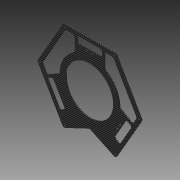
# Autodesk Inventor part: Bottom Plate
Saved by Autodesk Inventor 2015 (Build 190159000, 159)
## iProperties
Created: 2016-10-01
Part Number: Bottom Plate
Material: Generic
Document SubType Name: Modeling
Designer: James Yelland
Density: 1 g/cm^3
Appearance: Default
Author: James Yelland
Autodesk Inventor part; units mm, degrees
ref_plane "YZ Plane" through (0, 0, 0) normal (1, 0, 0) x (0, 1, 0)
ref_plane "XZ Plane" through (0, 0, 0) normal (0, 1, 0) x (-1, 0, 0)
ref_plane "XY Plane" through (0, 0, 0) normal (0, 0, 1) x (1, 0, 0)
sketch "Sketch1" plane through (0, 0, 0) normal (0, 1, 0) x (-1, 0, 0)
  line L0 (72.6878, -41.9663) -> (62.1878, -60.1529)
  line L1 (72.6878, -41.9663) -> (83.1878, -23.7798)
  line L2 (81.7237, -18.3157) -> (77.3936, -15.8157)
  line L3 (71.9295, -17.2797) -> (50.9295, -53.6529)
  line L4 (52.3936, -59.117) -> (56.7237, -61.617)
  arc A0 (56.7237, -61.617) -> (62.1878, -60.1529) centre (58.7237, -58.1529) ccw
  arc A1 (50.9295, -53.6529) -> (52.3936, -59.117) centre (54.3936, -55.6529) ccw
  arc A2 (77.3936, -15.8157) -> (71.9295, -17.2797) centre (75.3936, -19.2798) ccw
  arc A3 (83.1878, -23.7798) -> (81.7237, -18.3157) centre (79.7237, -21.7798) ccw
  line L5 (55.5994, -35.5644) -> (57.3314, -36.5644)
  line L6 (57.3314, -36.5644) -> (54.8314, -40.8945)
  line L7 (53.0994, -39.8945) -> (55.5994, -35.5644)
  line L8 (54.8314, -40.8945) -> (53.0994, -39.8945)
  line L9 (61.0994, -26.0381) -> (58.5994, -30.3683)
  line L10 (60.3314, -31.3683) -> (62.8314, -27.0381)
  line L11 (58.5994, -30.3683) -> (60.3314, -31.3683)
  line L12 (62.8314, -27.0381) -> (61.0994, -26.0381)
  line L13 (0, 83.9327) -> (21, 83.9327)
  line L14 (0, 83.9327) -> (-21, 83.9327)
  line L15 (-25, 79.9327) -> (-25, 74.9327)
  line L16 (-21, 70.9327) -> (20.9998, 70.9327)
  line L17 (25, 74.9327) -> (25, 79.9327)
  arc A4 (25, 79.9327) -> (21, 83.9327) centre (21, 79.9327) ccw
  arc A5 (20.9998, 70.9327) -> (25, 74.9327) centre (21, 74.9327) ccw
  arc A6 (-25, 74.9327) -> (-21, 70.9327) centre (-21, 74.9327) ccw
  arc A7 (-21, 83.9327) -> (-25, 79.9327) centre (-21, 79.9327) ccw
  line L18 (3, 65.9327) -> (3, 67.9327)
  line L19 (8, 65.9327) -> (3, 65.9327)
  line L20 (8, 67.9327) -> (8, 65.9327)
  line L21 (3, 67.9327) -> (8, 67.9327)
  line L22 (-8, 67.9327) -> (-8, 65.9327)
  line L23 (-8, 65.9327) -> (-3, 65.9327)
  line L24 (-3, 65.9327) -> (-3, 67.9327)
  line L25 (-3, 67.9327) -> (-8, 67.9327)
  line L26 (-72.6878, -41.9663) -> (-83.1878, -23.7798)
  line L27 (-72.6878, -41.9663) -> (-62.1878, -60.1529)
  line L28 (-56.7237, -61.617) -> (-52.3936, -59.117)
  line L29 (-50.9295, -53.6529) -> (-71.9294, -17.28)
  line L30 (-77.3936, -15.8157) -> (-81.7237, -18.3157)
  arc A8 (-81.7237, -18.3157) -> (-83.1878, -23.7798) centre (-79.7237, -21.7798) ccw
  arc A9 (-71.9294, -17.28) -> (-77.3936, -15.8157) centre (-75.3936, -19.2798) ccw
  arc A10 (-52.3936, -59.117) -> (-50.9295, -53.6529) centre (-54.3936, -55.6529) ccw
  arc A11 (-62.1878, -60.1529) -> (-56.7237, -61.617) centre (-58.7237, -58.1529) ccw
  line L31 (-58.5994, -30.3683) -> (-60.3314, -31.3683)
  line L32 (-61.0994, -26.0381) -> (-58.5994, -30.3683)
  line L33 (-62.8314, -27.0381) -> (-61.0994, -26.0381)
  line L34 (-60.3314, -31.3683) -> (-62.8314, -27.0381)
  line L35 (-54.8314, -40.8945) -> (-53.0994, -39.8945)
  line L36 (-53.0994, -39.8945) -> (-55.5994, -35.5644)
  line L37 (-55.5994, -35.5644) -> (-57.3314, -36.5644)
  line L38 (-57.3314, -36.5644) -> (-54.8314, -40.8945)
  line L39 (103.5566, -2.5) -> (54.8095, -86.9325)
  line L40 (-54.8095, -86.9325) -> (-103.5566, -2.5)
  line L41 (-103.5566, 2.5) -> (-53.9434, 88.4327)
  line L42 (-49.6132, 90.9327) -> (49.6132, 90.9327)
  line L43 (53.9434, 88.4327) -> (103.5566, 2.5)
  line L44 (2.1497, -66.9563) -> (48.3297, -88.9468)
  line L45 (-2.1497, -66.9563) -> (-48.3297, -88.9468)
  arc A12 (48.3297, -88.9468) -> (54.8095, -86.9325) centre (50.4794, -84.4325) ccw
  arc A13 (2.1497, -66.9563) -> (-2.1497, -66.9563) centre (0, -71.4706) ccw
  arc A14 (-54.8095, -86.9325) -> (-48.3297, -88.9468) centre (-50.4794, -84.4325) ccw
  arc A15 (-103.5566, 2.5) -> (-103.5566, -2.5) centre (-99.2265, 0) ccw
  arc A16 (-49.6132, 90.9327) -> (-53.9434, 88.4327) centre (-49.6132, 85.9327) ccw
  arc A17 (53.9434, 88.4327) -> (49.6132, 90.9327) centre (49.6132, 85.9327) ccw
  arc A18 (103.5566, -2.5) -> (103.5566, 2.5) centre (99.2265, 0) ccw
  circle A19 centre (49.6132, 85.9327) radius 1.6
  circle A20 centre (-49.6132, 85.9327) radius 1.6
  circle A21 centre (-99.2265, 0) radius 1.6
  circle A22 centre (99.2265, 0) radius 1.6
  line L46 (48.9434, 79.7724) -> (93.5566, 2.5)
  line L47 (-35, 82.2724) -> (-44.6132, 82.2724)
  line L48 (35, 82.2724) -> (44.6132, 82.2724)
  arc A23 (35, 82.2724) -> (30, 77.2724) centre (35, 77.2724) ccw
  arc A24 (-30, 77.2724) -> (-35, 82.2724) centre (-35, 77.2724) ccw
  arc A25 (48.9434, 79.7724) -> (44.6132, 82.2724) centre (44.6132, 77.2724) ccw
  line L49 (-93.5566, 2.5) -> (-48.9434, 79.7724)
  line L50 (-88.75, -10.8253) -> (-93.5566, -2.5)
  arc A26 (-88.75, -10.8253) -> (-81.9199, -12.6554) centre (-84.4199, -8.3253) ccw
  arc A27 (-93.5566, 2.5) -> (-93.5566, -2.5) centre (-89.2265, 0) ccw
  line L51 (88.75, -10.8253) -> (93.5566, -2.5)
  arc A28 (81.9199, -12.6554) -> (88.75, -10.8253) centre (84.4199, -8.3253) ccw
  arc A29 (-44.6132, 82.2724) -> (-48.9434, 79.7724) centre (-44.6132, 77.2724) ccw
  arc A30 (93.5566, -2.5) -> (93.5566, 2.5) centre (89.2265, 0) ccw
  line L52 (81.9199, -12.6554) -> (61.4758, -0.8521)
  line L53 (30, 77.2724) -> (30, 53.6656)
  line L54 (-30, 77.2724) -> (-30, 53.6656)
  line L55 (-81.9199, -12.6554) -> (-61.4758, -0.8521)
  circle A31 centre (0, 0) radius 47.5
  arc A32 (59.977, 1.6629) -> (31.4286, 51.1101) centre (0, 0) ccw
  arc A33 (-31.4286, 51.1101) -> (-59.977, 1.6629) centre (0, 0) ccw
  arc A34 (59.977, 1.6629) -> (61.4758, -0.8521) centre (62.9758, 1.746) ccw
  arc A35 (30, 53.6656) -> (31.4286, 51.1101) centre (33, 53.6656) ccw
  arc A36 (-31.4286, 51.1101) -> (-30, 53.6656) centre (-33, 53.6656) ccw
  arc A37 (-61.4758, -0.8521) -> (-59.977, 1.6629) centre (-62.9758, 1.746) ccw
  circle A38 centre (50.4794, -84.4325) radius 1.6
  circle A39 centre (-50.4794, -84.4325) radius 1.6
  circle A40 centre (0, 0) radius 53.75
  line L56 (-259.0503, -40.7163) -> (-260.5503, -40.7163)
  line L57 (-259.0503, -40.7163) -> (-257.5503, -40.7163)
  line L58 (-257.5503, -40.7163) -> (-257.5503, -43.7163)
  line L59 (-257.5503, -43.7163) -> (-254.5503, -43.7163)
  line L60 (-254.5503, -43.7163) -> (-254.5503, -37.7163)
  line L61 (-254.5503, -37.7163) -> (-257.5503, -37.7163)
  line L62 (-257.5503, -37.7163) -> (-257.5503, -40.7163)
  line L63 (-255.3646, -41.687) -> (-256.6146, -41.687)
  line L64 (-256.6146, -41.687) -> (-256.6146, -39.687)
  line L65 (-256.6146, -39.687) -> (-255.3646, -39.687)
  line L66 (-255.3646, -39.687) -> (-255.3646, -41.687)
  line L67 (-260.5503, -40.7163) -> (-260.5503, -43.7163)
  line L68 (-260.5503, -43.7163) -> (-263.5503, -43.7163)
  line L69 (-260.5503, -40.7163) -> (-260.5503, -40.7163)
  line L70 (-260.5503, -40.7163) -> (-260.5503, -37.7163)
  line L71 (-260.5503, -40.7163) -> (-257.5503, -40.7163) construction
  line L72 (-260.5503, -37.7163) -> (-263.5503, -37.7163)
  line L73 (-263.5503, -43.7163) -> (-263.5503, -37.7163)
  line L74 (-261.3995, -41.6595) -> (-262.1995, -41.6595)
  line L75 (-262.1995, -41.6595) -> (-262.1995, -39.9595)
  line L76 (-262.1995, -39.9595) -> (-261.3995, -39.9595)
  line L77 (-261.3995, -39.9595) -> (-261.3995, -41.6595)
  point P0 (60.1878, -63.617)
  point P1 (85.1878, -20.3157)
  point P2 (73.9295, -13.8157)
  point P3 (48.9295, -57.117)
  point P4 (25, 83.9327)
  point P5 (-25, 83.9327)
  point P6 (-25, 70.9327)
  point P7 (25, 70.9327)
  point P8 (-85.1878, -20.3157)
  point P9 (-60.1878, -63.617)
  point P10 (-48.9295, -57.117)
  point P11 (-73.9295, -13.8157)
  point P12 (105, 0)
  point P13 (52.5, -90.9327)
  point P14 (-105, 0)
  point P15 (-52.5, 90.9327)
  point P16 (52.5, 90.9327)
  point P17 (-86.25, -15.1554)
  point P18 (60, 0)
  point P19 (30, 51.9615)
  point P20 (-30, 51.9615)
  point P21 (-60, 0)
  dimension "d11" = 360
  dimension "d30" = 360
  dimension "d32" = 5
  dimension "d53" = 3
  dimension "d59" = 3.2
  dimension "d60" = 3.2
  dimension "d61" = 107.5
  dimension "d62" = 1.5
  dimension "d63" = 1.5
  dimension "d64" = 3
  dimension "d65" = 3
  dimension "d66" = 6
  dimension "d67" = 1.25
  dimension "d68" = 2
  dimension "d69" = 3
  dimension "d70" = 3
  dimension "d72" = 3
  dimension "d73" = 90
  dimension "d74" = 3
  dimension "d75" = 90
  dimension "d76" = 0.8
  dimension "d77" = 1.7
  constraints: 156 end point, 70 point on circle, 41 centre point, 40 point on line, 12 perpendicular, 12 tangent, 9 coincident, 6 horizontal, 4 equal radius, 4 vertical
  measures "d32" radius of A29
  measures "d53" radius of A34
  measures "d59" diameter of A38
  measures "d60" diameter of A39
  measures "d61" diameter of A40
  measures "d62" distance of L56.start L56.end
  measures "d63" distance of L56.start L57.end
  measures "d64" distance of L57.end L58.end
  measures "d65" distance of L58.end L59.end
  measures "d66" distance of L59.end L60.end
  measures "d67" distance of L63.start L63.end
  measures "d68" distance of L63.end L64.end
  measures "d69" distance of L56.end L67.end
  measures "d70" distance of L67.end L68.end
  measures "d72" distance of L69.start L70.end
  measures "d73" angle of L71 L70
  measures "d74" distance of L70.end L72.end
  measures "d75" angle of L72 L70
  measures "d76" distance of L77.end L75.start
  measures "d77" distance of L75.start L75.end
extrude "Extrusion1" add sketch "Sketch1" along normal blind 2 contours L39 A12 L44 A13 L45 A14 L40 A15 L41 A16 L42 A17 L43 A18 | A40
body "Solid1"
